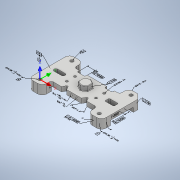
# Autodesk Inventor part: INV_nist_ctc_01_asme1_2021
Saved by Autodesk Inventor 2021 (Build 250183000, 183)
## iProperties
Created: 2016-11-24
Part Number: INV_nist_ctc_01_asme1_2021
Material: Generic
Document SubType Name: Modeling
Designer: t_liuje
Density: 1 g/cm^3
Appearance: Default
Author: t_liuje
Autodesk Inventor part; units mm, degrees
note: some values were not read from the file. Chosen so that the rebuilt part matches the saved one: direction of "Hole5".
ref_plane "YZ Plane" through (0, 0, 0) normal (1, 0, 0) x (0, 1, 0)
ref_plane "XZ Plane" through (0, 0, 0) normal (0, 1, 0) x (-1, 0, 0)
ref_plane "XY Plane" through (0, 0, 0) normal (0, 0, 1) x (1, 0, 0)
sketch "NLST  LOGO" plane through (0, 0, 0) normal (0, 0, 1) x (1, 0, 0)
  line L0 (31.5439, 94.2591) -> (15.3375, 94.2591)
  arc A0 (31.5439, 94.2591) -> (37.8375, 100.5528) centre (31.5439, 100.5528) ccw
  line L1 (37.8375, 123.3535) -> (37.8375, 100.5528)
  arc A1 (37.8375, 123.3535) -> (24.3031, 123.3535) centre (31.0703, 122.2758) ccw
  line L2 (24.3031, 108.9133) -> (24.3031, 123.3535)
  arc A2 (20.079, 109.0858) -> (24.3031, 108.9133) centre (22.1875, 108.9133) ccw
  line L3 (20.079, 132.6209) -> (20.079, 109.0858)
  line L4 (37.8375, 132.6209) -> (20.079, 132.6209)
  line L5 (37.8375, 137.2747) -> (37.8375, 132.6209)
  line L6 (20.079, 137.2747) -> (37.8375, 137.2747)
  line L7 (20.079, 146.8886) -> (20.079, 137.2747)
  line L8 (15.3375, 146.8886) -> (20.079, 146.8886)
  line L9 (15.3375, 108.4837) -> (15.3375, 146.8886)
  arc A3 (15.3375, 108.4837) -> (28.9581, 108.9996) centre (22.1576, 108.4837) ccw
  line L10 (28.9581, 122.5773) -> (28.9581, 108.9996)
  arc A4 (33.1827, 122.6636) -> (28.9581, 122.5773) centre (31.0751, 122.3933) ccw
  line L11 (33.1827, 100.5964) -> (33.1827, 122.6636)
  arc A5 (31.5439, 98.9575) -> (33.1827, 100.5964) centre (31.5439, 100.5964) ccw
  line L12 (15.3375, 98.9575) -> (31.5439, 98.9575)
  line L13 (15.3375, 94.2591) -> (15.3375, 98.9575)
  line L14 (37.8375, 61.5875) -> (19.5944, 61.5875)
  line L15 (37.8375, 66.2412) -> (37.8375, 61.5875)
  line L16 (20.9723, 66.2412) -> (37.8375, 66.2412)
  arc A6 (20.424, 67.647) -> (20.9723, 66.2412) centre (20.9723, 67.051) ccw
  line L17 (35.8584, 81.8477) -> (20.424, 67.647)
  arc A7 (35.8584, 81.8477) -> (32.5618, 91.2424) centre (32.5618, 85.9667) ccw
  line L18 (15.3375, 91.2424) -> (32.5618, 91.2424)
  line L19 (15.3375, 86.544) -> (15.3375, 91.2424)
  line L20 (32.4497, 86.544) -> (15.3375, 86.544)
  arc A8 (32.924, 85.4676) -> (32.4497, 86.544) centre (32.5018, 85.9242) ccw
  line L21 (16.2734, 70.0703) -> (32.924, 85.4676)
  arc A9 (16.2734, 70.0703) -> (19.5944, 61.5875) centre (19.5944, 66.479) ccw
sketch "Block2" plane through (0, 0, 0) normal (0, 0, 1) x (1, 0, 0)
  line L0 (22.7156, 121.766) -> (22.7156, 107.3258)
  line L1 (27.3706, 107.4121) -> (27.3706, 120.9898)
  line L2 (31.5952, 121.0761) -> (31.5952, 99.0089)
  line L3 (29.9564, 97.37) -> (13.75, 97.37)
  arc A0 (29.9564, 92.6716) -> (36.25, 98.9653) centre (29.9564, 98.9653) ccw
  line L4 (13.75, 92.6716) -> (29.9564, 92.6716)
  line L5 (13.75, 97.37) -> (13.75, 92.6716)
  arc A1 (18.4915, 107.4983) -> (22.7156, 107.3258) centre (20.6, 107.3258) ccw
  arc A2 (31.5952, 121.0761) -> (27.3706, 120.9898) centre (29.4876, 120.8058) ccw
  arc A3 (36.25, 121.766) -> (22.7156, 121.766) centre (29.4828, 120.6883) ccw
  line L6 (18.4915, 131.0334) -> (36.25, 131.0334)
  line L7 (18.4915, 107.4983) -> (18.4915, 131.0334)
  line L8 (13.75, 145.3011) -> (13.75, 106.8962)
  line L9 (36.25, 131.0334) -> (36.25, 135.6872)
  line L10 (36.25, 135.6872) -> (18.4915, 135.6872)
  line L11 (18.4915, 145.3011) -> (13.75, 145.3011)
  line L12 (18.4915, 135.6872) -> (18.4915, 145.3011)
  line L13 (36.25, 98.9653) -> (36.25, 121.766)
  arc A4 (13.75, 106.8962) -> (27.3706, 107.4121) centre (20.5701, 106.8962) ccw
  arc A5 (29.9564, 97.37) -> (31.5952, 99.0089) centre (29.9564, 99.0089) ccw
  line L14 (18.0069, 60) -> (36.25, 60)
  arc A6 (14.6859, 68.4828) -> (18.0069, 60) centre (18.0069, 64.8915) ccw
  line L15 (31.3365, 83.8801) -> (14.6859, 68.4828)
  arc A7 (31.3365, 83.8801) -> (30.8622, 84.9565) centre (30.9143, 84.3367) ccw
  line L16 (13.75, 84.9565) -> (30.8622, 84.9565)
  line L17 (13.75, 89.6549) -> (13.75, 84.9565)
  line L18 (30.9743, 89.6549) -> (13.75, 89.6549)
  arc A8 (34.2709, 80.2602) -> (30.9743, 89.6549) centre (30.9743, 84.3792) ccw
  arc A9 (18.8365, 66.0595) -> (19.3848, 64.6537) centre (19.3848, 65.4635) ccw
  line L19 (36.25, 64.6537) -> (19.3848, 64.6537)
  line L20 (36.25, 60) -> (36.25, 64.6537)
  line L21 (18.8365, 66.0595) -> (34.2709, 80.2602)
  point P0 (24.9635, 99.9518)
sketch "Sketch1" plane through (0, 0, 0) normal (0, 0, 1) x (1, 0, 0)
  line L0 (0, 0) -> (0, 450)
  line L1 (0, 450) -> (150, 450)
  line L2 (150, 450) -> (150, 350)
  line L3 (650, 450) -> (800, 450)
  line L4 (800, 450) -> (800, 0)
  line L5 (800, 0) -> (650, 0)
  line L6 (650, 0) -> (650, 100)
  line L7 (150, 100) -> (150, 0)
  line L8 (150, 0) -> (0, 0)
  line L9 (150, 350) -> (207.5, 350)
  line L10 (207.5, 350) -> (207.5, 325)
  line L11 (207.5, 325) -> (292.5, 325)
  line L12 (292.5, 325) -> (292.5, 350)
  line L13 (292.5, 350) -> (507.5, 350)
  line L14 (507.5, 350) -> (507.5, 325)
  line L15 (507.5, 325) -> (592.5, 325)
  line L16 (592.5, 325) -> (592.5, 350)
  line L17 (592.5, 350) -> (650, 350)
  line L18 (650, 350) -> (650, 450)
  line L19 (650, 100) -> (538.8675, 100)
  line L20 (538.8675, 100) -> (510, 150)
  line L21 (510, 150) -> (481.1325, 100)
  line L22 (481.1325, 100) -> (318.8675, 100)
  line L23 (318.8675, 100) -> (290, 150)
  line L24 (290, 150) -> (261.1325, 100)
  line L25 (261.1325, 100) -> (150, 100)
  dimension "d8" = 450
  dimension "d9" = 150
  dimension "d10" = 100
  dimension "d13" = 150
  dimension "d14" = 150
  dimension "d15" = 100
  dimension "d16" = 150
  dimension "d19" = 57.5
  dimension "d20" = 25
  dimension "d21" = 85
  dimension "d25" = 215
  dimension "d26" = 85
  dimension "d27" = 25
  dimension "d28" = 25
  dimension "d29" = 57.5
  dimension "d30" = 25
  dimension "d36" = 140
  dimension "d37" = 120
  dimension "d38" = 50
  dimension "d39" = 60
  dimension "d40" = 140
  dimension "d41" = 60
  dimension "d42" = 60
  dimension "d43" = 50
  constraints: 52 end point, 11 perpendicular, 5 horizontal, 4 point on line, 3 vertical, 2 collinear
  measures "d8" distance of L0.start L0.end
  measures "d9" distance of L0.end L1.end
  measures "d10" distance of L1.end L2.end
  measures "d13" distance of L3.start L3.end
  measures "d14" distance of L4.end L5.end
  measures "d15" distance of L5.end L6.end
  measures "d16" distance between parallel lines of L0 L7
  measures "d19" distance of L2.end L9.end
  measures "d20" distance of L9.end L10.end
  measures "d21" distance of L10.end L11.end
  measures "d25" distance of L12.end L13.end
  measures "d26" distance of L14.end L15.end
  measures "d27" distance of L11.end L12.end
  measures "d28" distance of L13.end L14.end
  measures "d29" distance of L16.end L17.end
  measures "d30" distance of L15.end L16.end
  measures "d36" distance from line of L6 L20.end
  measures "d37" angle of L19 L20
  measures "d38" distance from line of L19 L20.end
  measures "d39" angle of L22 L21
  measures "d40" distance from line of L7 L23.end
  measures "d41" angle of L25 L24
  measures "d42" angle of L22 L23
  measures "d43" distance from line of L25 L23.end
extrude "Extrusion1" add sketch "Sketch1" against normal blind 50
sketch "Sketch2" plane through (0, 0, -50) normal (0, 0, -1) x (-1, 0, 0)
  line L0 (-650, 100) -> (-538.8675, 100) projected
  line L1 (-800, 0) -> (-650, 0) projected
  line L2 (-650, 100) -> (-800, 100)
  line L3 (-800, 100) -> (-800, 0)
  line L4 (-800, 0) -> (-650, 0)
  line L5 (-650, 0) -> (-650, 100)
  line L6 (-150, 100) -> (-150, 0) projected
  line L7 (-150, 100) -> (0, 100)
  line L8 (0, 100) -> (0, 0)
  line L9 (0, 0) -> (-150, 0)
  line L10 (-150, 0) -> (-150, 100)
  line L11 (-150, 350) -> (-207.5, 350) projected
  line L12 (0, 0) -> (0, 450) projected
  line L13 (-150, 350) -> (0, 350)
  line L14 (0, 350) -> (0, 450)
  line L15 (0, 450) -> (-150, 450)
  line L16 (-150, 450) -> (-150, 350)
  line L17 (-650, 350) -> (-650, 450) projected
  line L18 (-800, 450) -> (-800, 0) projected
  line L19 (-650, 350) -> (-800, 350)
  line L20 (-800, 350) -> (-800, 450)
  line L21 (-800, 450) -> (-650, 450)
  line L22 (-650, 450) -> (-650, 350)
  constraints: 32 end point, 8 parallel, 4 horizontal, 4 perpendicular
extrude "Extrusion2" add sketch "Sketch2" along normal blind 50
fillet "Fillet1" radius 50 7 edges at (0, 450, -50) (0, 0, -50) (800, 0, -50) (150, 0, -50) (650, 0, -50) (150, 450, -50) (650, 450, -50)
fillet "Fillet2" radius 25 4 edges at (150, 100, -25) (650, 100, -25) (150, 350, -25) (650, 350, -25)
chamfer "Chamfer1" distance 50 angle 45 1 edges at (800, 450, -50)
fillet "Fillet3" radius 10 14 edges at (207.5, 325, -25) (507.5, 325, -25) (292.5, 325, -25) (592.5, 325, -25) (290, 150, -25) (510, 150, -25) (75, 100, -50) (150, 87.5, -50) (150, 362.5, -50) (75, 350, -50) (725, 100, -50) (650, 87.5, -50) (650, 362.5, -50) (725, 350, -50)
sketch "Sketch3" plane through (0, 0, 0) normal (0, 0, 1) x (1, 0, 0)
  line L0 (350, 253.8675) -> (400, 282.735)
  line L1 (400, 282.735) -> (450, 253.8675)
  line L2 (450, 253.8675) -> (450, 196.1325)
  line L3 (450, 196.1325) -> (400, 167.265)
  line L4 (400, 167.265) -> (350, 196.1325)
  line L5 (350, 196.1325) -> (350, 253.8675)
  line L6 (0, 50) -> (0, 400) projected
  line L7 (292.5, 350) -> (507.5, 350) projected
  point P0 (0, 0)
  point P1 (400, 225)
  dimension "d88" = 400
  dimension "d89" = 125
  dimension "d90" = 50
  constraints: 12 end point, 1 vertical, 13 other
  measures "d88" distance from line of L6 point (400, 225)
  measures "d89" distance from line of point (400, 225) L7
  measures "d90" distance from line of L5 point (400, 225)
extrude "Extrusion3" add sketch "Sketch3" along normal blind 50
fillet "Fillet4" radius 5 6 edges at (425, 181.6987, 0) (450, 225, 0) (425, 268.3013, 0) (375, 268.3013, 0) (350, 225, 0) (375, 181.6987, 0)
chamfer "Chamfer2" distance 5 angle 45 6 edges at (425, 181.6987, 50) (450, 225, 50) (425, 268.3013, 50) (375, 268.3013, 50) (350, 225, 50) (375, 181.6987, 50)
hole "Hole1" at (75, 400, 0) direction (0, 0, -1) diameter 35 end through all
hole "Hole2" at (75, 50, 0) direction (0, 0, -1) diameter 35 end through all
hole "Hole3" at (725, 50, 0) direction (0, 0, -1) diameter 35 end through all
hole "Hole4" at (725, 400, 0) direction (0, 0, -1) diameter 35 end through all
sketch "Sketch4" plane through (0, 0, 0) normal (0, 0, 1) x (1, 0, 0)
  line L0 (75, 245) -> (155, 245)
  line L1 (155, 205) -> (75, 205)
  line L2 (50, 450) -> (100, 450) projected
  line L3 (0, 50) -> (0, 400) projected
  arc A0 (155, 205) -> (155, 245) centre (155, 225) ccw
  arc A1 (75, 245) -> (75, 205) centre (75, 225) ccw
  line L4 (645, 250) -> (725, 250)
  line L5 (735, 240) -> (735, 210)
  line L6 (725, 200) -> (645, 200)
  line L7 (635, 210) -> (635, 240)
  line L8 (700, 450) -> (750, 450) projected
  line L9 (800, 400) -> (800, 50) projected
  arc A2 (645, 250) -> (635, 240) centre (645, 240) ccw
  arc A3 (635, 210) -> (645, 200) centre (645, 210) ccw
  arc A4 (725, 200) -> (735, 210) centre (725, 210) ccw
  arc A5 (735, 240) -> (725, 250) centre (725, 240) ccw
  point P0 (0, 0)
  point P1 (735, 200)
  point P2 (735, 250)
  point P3 (635, 200)
  dimension "d97" = 80
  dimension "d98" = 40
  dimension "d99" = 205
  dimension "d101" = 75
  dimension "d102" = 100
  dimension "d103" = 50
  dimension "d104" = 200
  dimension "d105" = 65
  dimension "d106" = 10
  constraints: 12 end point, 12 point on circle, 12 tangent, 6 centre point, 6 point on line, 3 equal radius, 3 parallel, 2 horizontal, 1 perpendicular
  measures "d97" distance of L1.start L1.end
  measures "d98" distance of L0.end L1.start
  measures "d99" distance between parallel lines of L0 L2
  measures "d101" distance from line of L3 A1.centre
  measures "d102" distance of point (735, 200) point (635, 200)
  measures "d103" distance of point (735, 250) point (735, 200)
  measures "d104" distance between parallel lines of L4 L8
  measures "d105" distance between parallel lines of L9 L5
  measures "d106" radius of A2
extrude "Extrusion4" cut sketch "Sketch4" against normal up to surface (50 mm away)
hole "Hole5" at (240, 180, 0) direction (0, 0, -1) diameter 25 end up to surface
pattern_linear "Rectangular Pattern1" count 2 spacing 90 along (0, 1, 0) count 2 spacing 320 along (1, 0, 0) of "Hole5"
hole "Hole6" at (370, 100, -25) direction (0, 1, 0) diameter 20 depth 45 tip angle 118
hole "Hole7" at (430, 100, -25) direction (0, 1, 0) diameter 20 depth 45 tip angle 118
sketch "Sketch5" plane through (800, 50, -100) normal (1, 0, 0) x (0, 0, -1)
  line L0 (0, 0) -> (-100, 0) projected
  line L1 (-50, 290) -> (-50, 60) projected
  line L2 (-77.2844, 121.766) -> (-77.2844, 107.3258)
  line L3 (-72.6294, 107.4121) -> (-72.6294, 120.9898)
  line L4 (-68.4048, 121.0761) -> (-68.4048, 99.0089)
  line L5 (-70.0436, 97.37) -> (-86.25, 97.37)
  arc A0 (-70.0436, 92.6716) -> (-63.75, 98.9653) centre (-70.0436, 98.9653) ccw
  line L6 (-86.25, 92.6716) -> (-70.0436, 92.6716)
  line L7 (-86.25, 97.37) -> (-86.25, 92.6716)
  arc A1 (-81.5085, 107.4983) -> (-77.2844, 107.3258) centre (-79.4, 107.3258) ccw
  arc A2 (-68.4048, 121.0761) -> (-72.6294, 120.9898) centre (-70.5124, 120.8058) ccw
  arc A3 (-63.75, 121.766) -> (-77.2844, 121.766) centre (-70.5172, 120.6883) ccw
  line L8 (-81.5085, 131.0334) -> (-63.75, 131.0334)
  line L9 (-81.5085, 107.4983) -> (-81.5085, 131.0334)
  line L10 (-86.25, 145.3011) -> (-86.25, 106.8962)
  line L11 (-63.75, 131.0334) -> (-63.75, 135.6872)
  line L12 (-63.75, 135.6872) -> (-81.5085, 135.6872)
  line L13 (-81.5085, 145.3011) -> (-86.25, 145.3011)
  line L14 (-81.5085, 135.6872) -> (-81.5085, 145.3011)
  line L15 (-63.75, 98.9653) -> (-63.75, 121.766)
  arc A4 (-86.25, 106.8962) -> (-72.6294, 107.4121) centre (-79.4299, 106.8962) ccw
  arc A5 (-70.0436, 97.37) -> (-68.4048, 99.0089) centre (-70.0436, 99.0089) ccw
  line L16 (-81.9931, 60) -> (-63.75, 60)
  arc A6 (-85.3141, 68.4828) -> (-81.9931, 60) centre (-81.9931, 64.8915) ccw
  line L17 (-68.6635, 83.8801) -> (-85.3141, 68.4828)
  arc A7 (-68.6635, 83.8801) -> (-69.1378, 84.9565) centre (-69.0857, 84.3367) ccw
  line L18 (-86.25, 84.9565) -> (-69.1378, 84.9565)
  line L19 (-86.25, 89.6549) -> (-86.25, 84.9565)
  line L20 (-69.0257, 89.6549) -> (-86.25, 89.6549)
  arc A8 (-65.7291, 80.2602) -> (-69.0257, 89.6549) centre (-69.0257, 84.3792) ccw
  arc A9 (-81.1635, 66.0595) -> (-80.6152, 64.6537) centre (-80.6152, 65.4635) ccw
  line L21 (-63.75, 64.6537) -> (-80.6152, 64.6537)
  line L22 (-63.75, 60) -> (-63.75, 64.6537)
  line L23 (-81.1635, 66.0595) -> (-65.7291, 80.2602)
  point P0 (-100, -50)
  dimension "d279" = 13.75
  dimension "d280" = 60
extrude "Extrusion5" cut sketch "Sketch5" against normal blind 2
equation "\"d27\" = d20"
equation "\"d28\" = d27"
equation "\"d29\" = d19"
equation "\"d40\" = d36"
equation "\"d41\" = d39"
equation "\"d42\" = d39"
equation "\"d43\" = d38"
body "Solid1"
